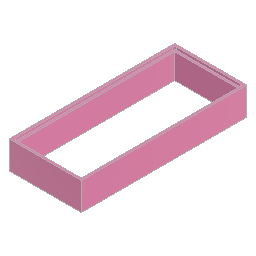
Dry-Erase-Marker-Holder (Autodesk Fusion 360 design; units mm, degrees)
Autodesk Fusion 360 part; units mm, degrees
sketch "Sketch1" plane through (0, 0, 3.175) normal (0, 0, 1) x (-1, 0, 0)
  line L0 (0, 0) -> (0, 297.942)
  line L1 (0, 297.942) -> (-407.924, 297.942)
  line L2 (-407.924, 297.942) -> (-407.924, 0)
  line L3 (-407.924, 0) -> (0, 0)
  line L4 (-51.1, 148.972) -> (0, 148.972)
  line L5 (-134.55, 148.972) -> (-51.1, 148.972)
  line L6 (0, 0) -> (-65, 0)
  line L7 (-65, 0) -> (-65, 148.972)
  line L8 (-65, 148.972) -> (0, 148.972)
  line L9 (0, 148.972) -> (0, 0)
  line L10 (-4, 144.972) -> (-4, 4)
  line L11 (-4, 4) -> (-61, 4)
  line L12 (-61, 4) -> (-61, 144.972)
  line L13 (-61, 144.972) -> (-4, 144.972)
  dimension "d188" = 148.972
  dimension "d189" = 65
  dimension "d190" = 4
  constraint horizontal L6
  constraint vertical L7
  constraint horizontal L8
  constraint vertical L9
  constraint coincident L5 L7.end
  constraint coincident L0.start L3.end
  measures "d188" distance of L0.start L4.end
  measures "d189" distance of L0.start L6.end
extrude "Extrude1" add sketch "Sketch1" along normal blind 25 contours L0 L3 L4 L5 L6 L7 L8 L9
sketch "Sketch2" plane through (0, 0, 28.175) normal (0, 0, 1) x (-1, 0, 0)
  line L0 (-61, 4) -> (-61, 144.972)
  line L1 (-61, 144.972) -> (-4, 144.972)
  line L2 (-4, 144.972) -> (-4, 4)
  line L3 (-4, 4) -> (-61, 4)
  line L4 (0, 148.972) -> (-65, 148.972)
  line L5 (-65, 148.972) -> (-65, 0)
  line L6 (-65, 0) -> (0, 0)
  line L7 (0, 0) -> (0, 148.972)
  line L8 (-2, 144.972) -> (-2, 4)
  line L9 (-4, 2) -> (-61, 2)
  line L10 (-63, 4) -> (-63, 144.972)
  line L11 (-61, 146.972) -> (-4, 146.972)
  arc A0 (-61, 146.972) -> (-63, 144.972) centre (-61, 144.972) ccw
  arc A1 (-63, 4) -> (-61, 2) centre (-61, 4) ccw
  arc A2 (-4, 2) -> (-2, 4) centre (-4, 4) ccw
  arc A3 (-2, 144.972) -> (-4, 146.972) centre (-4, 144.972) ccw
  dimension "d194" = 2
  constraint tangent L11 A0
  constraint tangent L10 A0
  constraint tangent L10 A1
  constraint tangent L9 A1
  constraint equal A0 A1
  constraint tangent L9 A2
  constraint tangent L8 A2
  constraint equal A0 A2
  constraint tangent L8 A3
  constraint tangent L11 A3
  constraint equal A0 A3
  measures "d194" radius of A0
extrude "Extrude2" cut sketch "Sketch2" against normal blind 2.5 contours L8 L9 L10 L11 A0 A1 A2 A3
equation "d190 = ComponentWallWidth"
equation "ComponentWallWidth = 4 mm"
